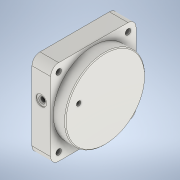
# Autodesk Inventor part: Deckel_hinten
Saved by Autodesk Inventor 2020.3 (Build 243373000, 373)
## iProperties
Created: 2021-05-20
Part Number: Deckel_hinten
Material: Stahl AISI 4130
Document SubType Name: Modeling
Designer: Preuß P. Ch.
Density: 7.85 g/cm^3
Appearance: Stahl
Author: Preuß P. Ch.
Autodesk Inventor part; units mm, degrees
ref_plane "YZ Plane" through (0, 0, 0) normal (1, 0, 0) x (0, 1, 0)
ref_plane "XZ Plane" through (0, 0, 0) normal (0, 1, 0) x (-1, 0, 0)
ref_plane "XY Plane" through (0, 0, 0) normal (0, 0, 1) x (1, 0, 0)
sketch "Skizze1" plane through (0, 0, 0) normal (0, 0, 1) x (1, 0, 0)
  line L0 (0, 80) -> (35, 80)
  line L1 (35, 80) -> (35, -80)
  line L2 (35, -80) -> (0, -80)
  line L3 (0, -80) -> (0, 80)
  line L4 (35, 75) -> (57.5, 75)
  line L5 (57.5, 75) -> (57.5, 0)
  line L6 (57.5, 0) -> (35, 0)
  line L7 (35, 0) -> (35, 75)
  point P0 (0, 0)
  point P1 (0, 0)
  dimension "d0" = 160
  dimension "d1" = 150
  dimension "d2" = 57.5
  dimension "d3" = 35
  constraints: 16 end point, 4 parallel, 2 horizontal, 2 perpendicular, 2 point on line, 1 coincident, 1 midpoint
  measures "d0" diameter of L0 L6
  measures "d1" diameter of L4 L6
  measures "d2" distance between parallel lines of L5 L3
  measures "d3" distance between parallel lines of L1 L3
extrude "Extrusion1" add sketch "Skizze1" along normal mid plane 160 contours L0 L1 L2 L3
revolve "Umdrehung1" add sketch "Skizze1" angle 360 about axis through (57.5, 0, 0) along (-1, 0, 0) contours L4 L5 L6 L1
fillet "Rundung1" radius 15 4 edges at (17.5, 80, 80) (17.5, 80, -80) (17.5, -80, 80) (17.5, -80, -80)
sketch "Skizze2" plane through (35, -65, -80) normal (1, 0, 0) x (0, 0, -1)
  line L0 (-15, 0) -> (-145, 0)
  line L1 (-145, 0) -> (-145, 130)
  line L2 (-145, 130) -> (-15, 130)
  line L3 (-15, 130) -> (-15, 0)
  line L4 (-15, 0) -> (-145, 130) construction
  line L5 (-145, 0) -> (-15, 130) construction
  point P0 (-80, 65)
  dimension "d8" = 130
  dimension "d9" = 130
  constraints: 12 end point, 2 midpoint, 2 parallel, 1 horizontal, 1 perpendicular
  measures "d8" distance of L1.end L2.end
  measures "d9" distance of L0.end L1.end
hole "Bohrung1" at (35, 65, 65) at (35, 65, -65) at (35, -65, 65) at (35, -65, -65) direction (-1, 0, 0) diameter 10.5 end through all
sketch "Skizze3" plane through (0, 0, 80) normal (0, 0, 1) x (1, 0, 0)
  line L0 (35, 80) -> (0, 80) projected
  line L1 (0, 65) -> (0, -65) projected
  point P0 (0, 0)
  point P1 (17.5, 17.5)
  dimension "d17" = 62.5
  dimension "d18" = 17.5
  measures "d17" distance from line of L0 point (17.5, 17.5)
  measures "d18" distance from line of L1 point (17.5, 17.5)
hole "Bohrung2" at (17.5, 17.5, 80) direction (0, 0, -1) diameter 8.376 depth 34.5 tip angle 118 counterbore diameter 20 counterbore depth 1.5 thread size "M10x1.5" class "6H" standard "ISO Metric profile"
sketch "Skizze4" plane through (57.5, 0, 0) normal (1, 0, 0) x (0, 0, -1)
  line L0 (-80, -65) -> (-80, 65) projected
  line L1 (65, 80) -> (-65, 80) projected
  point P0 (0, 0)
  point P1 (-50, 17.5)
  dimension "d26" = 30
  dimension "d27" = 62.5
  measures "d26" distance from line of L0 point (-50, 17.5)
  measures "d27" distance from line of L1 point (-50, 17.5)
hole "Bohrung3" at (57.5, 17.5, 50) direction (-1, 0, 0) diameter 8.5 depth 40 tip angle 118
chamfer "Fase1" distance 2 angle 45 1 edges at (17.5, 21.688, 78.5)
chamfer "Fase2" distance 1.5 angle 45 1 edges at (57.5, -75, 0)
equation "\"d4\" = d0"
